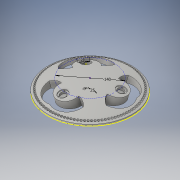
# Autodesk Inventor part: BB-8_headslider_dome
Saved by Autodesk Inventor 2016 (Build 200138000, 138)
## iProperties
Created: 2018-07-20
Part Number: BB-8_headslider_dome
Material: Generic
Document SubType Name: Modeling
Designer: Karcsi
Density: 1 g/cm^3
Appearance: Default
Author: Karcsi
Autodesk Inventor part; units mm, degrees
sketch "Sketch1" plane through (0, 0, 0) normal (0, 0, 1) x (1, 0, 0)
  arc A0 (0, 254) -> (-118.0215, 224.9154) centre (0, 0) ccw construction
  arc A1 (0, -254) -> (118.0215, 224.9154) centre (0, 0) ccw construction
  line L0 (0, 0) -> (0, 254)
  line L1 (0, 0) -> (0, -254)
  line L2 (-118.0215, 224.9154) -> (0, 224.9154) construction
  arc A2 (-118.0215, 224.9154) -> (0, -254) centre (0, 0) ccw construction
  arc A3 (118.0215, 224.9154) -> (0, 254) centre (0, 0) ccw
  line L3 (0, 224.9154) -> (88.5815, 224.9154) construction
  line L4 (0, 254) -> (0, 224.9154)
  line L5 (101.3234, 224.9154) -> (118.0215, 224.9154) construction
  line L6 (88.5815, 224.9154) -> (101.3234, 224.9154) construction
  line L7 (118.0215, 220.9154) -> (0, 220.9154)
  line L8 (0, 224.9154) -> (0, 220.9154)
  line L9 (118.0215, 224.9154) -> (118.0215, 220.9154)
  dimension "d0" = 508
  dimension "d1" = 236.043
  dimension "d23" = 4
  constraints: 20 end point, 8 point on circle, 4 centre point, 4 horizontal, 3 collinear, 2 point on line, 1 coincident, 1 parallel, 1 perpendicular, 1 vertical
  measures "d0" diameter of A0
  measures "d1" distance of L2.start L5.end
  measures "d23" distance between parallel lines of L3 L7
revolve "Revolution1" add sketch "Sketch1" angle 360 about axis through (0, 0, 0) along (0, 1, 0)
sketch "Sketch8" plane through (0, 220.9154, 0) normal (0, -1, 0) x (1, 0, 0)
  circle A0 centre (0, 0) radius 118.0215 projected
  line L0 (-84.745, -82.1423) -> (-100.1458, -62.4492)
  dimension "d24" = 25
  constraints: 2 end point, 2 point on circle
  measures "d24" distance of L0.start L0.end
ref_plane "Work Plane4" through (-86.2431, 224.9938, -83.3138) normal (0.3329064, -0.9063078, 0.2603451) x (-0.6160289, 0, 0.7877236)
ref_plane "Work Plane3" through (-84.745, 220.9154, -82.1423) normal (0.3329064, -0.9063078, 0.2603451) x (-0.6160289, 0, 0.7877236)
ref_plane "Work Plane5" through (0, 254.2529, 0) normal (0, -1, 0) x (1, 0, 0)
sketch "Sketch10" plane through (-86.2431, 224.9938, -83.3138) normal (0.3329064, -0.9063078, 0.2603451) x (-0.6160289, 0, 0.7877236)
  line L0 (9.3666, -17.4194) -> (9.0029, -1.1358) construction
  ellipse E0 centre (12.5, -108.0527) end of major axis (130.5215, -108.0527) minor radius 106.9638 projected
  circle A0 centre (9.1847, -9.2776) radius 2.75
  point P0 (12.5, -12.9993)
  dimension "d31" = 16.2836
  dimension "d32" = 5.5
  constraints: 2 end point, 1 centre point, 1 midpoint, 2 other
  measures "d31" vertical distance of L0.start L0.end
  measures "d32" diameter of A0
extrude "Extrusion6" cut sketch "Sketch10" along normal blind 8 contours A0
pattern_circular "Circular Pattern1" count 100 over 360 about axis through (0, -10, 0) along (0, 1, 0) of "Extrusion6"
ref_plane "Work Plane7" through (-86.8858, 231.0576, -83.8164) normal (0.2038779, -0.9659258, 0.15944) x (-0.6160289, 0, 0.7877236)
ref_plane "Work Plane6" through (-84.745, 220.9154, -82.1423) normal (0.2038779, -0.9659258, 0.15944) x (-0.6160289, 0, 0.7877236)
sketch "Sketch15" plane through (0, 254.2529, 0) normal (0, -1, 0) x (1, 0, 0)
  circle A0 centre (0, 0) radius 70 construction
  dimension "d43" = 140
  constraints: 1 centre point, 1 coincident
  measures "d43" diameter of A0
sketch "Sketch16" plane through (-86.8858, 231.0576, -83.8164) normal (0.2038779, -0.9659258, 0.15944) x (-0.6160289, 0, 0.7877236)
  ellipse E0 centre (12.5, -121.9872) end of major axis (82.5, -121.9872) minor radius 67.6148 projected
  line L0 (12.5, -298.4228) -> (12.5, 63.3053)
  line L1 (12.5, -258.4808) -> (-169.7544, -258.4808)
  line L2 (12.5, -258.4808) -> (193.6614, -258.4808)
  circle A0 centre (12.5, -54.3724) radius 12.5
  point P0 (12.5, -56.1817)
  dimension "d44" = 182.2544
  dimension "d45" = 181.1614
  dimension "d46" = 25
  constraints: 6 end point, 2 horizontal, 2 point on line, 1 centre point, 1 vertical, 1 vertical alignment, 1 other
  measures "d44" distance of L1.start L1.end
  measures "d45" distance of L1.start L2.end
  measures "d46" diameter of A0
sketch "Sketch17" plane through (-86.8858, 231.0576, -83.8164) normal (0.2038779, -0.9659258, 0.15944) x (-0.6160289, 0, 0.7877236)
  circle A0 centre (12.5, -54.3724) radius 8.5
  point P0 (12.5, -56.1817)
  dimension "d47" = 17
  constraints: 1 centre point, 1 coincident
  measures "d47" diameter of A0
extrude "Extrusion7" cut sketch "Sketch16" along normal blind 3 contours A0 L0 E0 | E0 L0 A0 | L0 A0 E0 | E0 A0 L0 picked at (13.5203, -62.5789) picked at (14.4702, -50.3327) picked at (11.4797, -62.5789) picked at (10.4798, -50.3445)
extrude "Extrusion8" cut sketch "Sketch17" along normal blind 9
pattern_circular "Circular Pattern2" count 3 over 360 about axis through (0, -10, 0) along (0, 1, 0) of "Extrusion8", "Extrusion7"
sketch "Sketch18" plane through (-52.6035, 242.2324, -41.1379) normal (-0.2038779, 0.9659258, -0.15944) x (0.9784424, 0.2065197, 0)
  point P0 (1.4437, -1.0906)
sketch "Sketch20" plane through (0, 220.9154, 0) normal (0, -1, 0) x (1, 0, 0)
  line L0 (12.5, 4.5) -> (-12.5, 4.5)
  line L1 (-12.5, 4.5) -> (-12.5, -4.5)
  line L2 (-12.5, -4.5) -> (12.5, -4.5)
  line L3 (12.5, -4.5) -> (12.5, 4.5)
  point P0 (0, 0)
  dimension "d60" = 25
  dimension "d61" = 9
  constraints: 8 end point, 2 parallel, 1 horizontal, 1 perpendicular
  measures "d60" distance of L2.end L1.end
  measures "d61" distance of L1.end L0.end
sketch "Sketch21" plane through (0, 220.9154, 0) normal (0, -1, 0) x (1, 0, 0)
  line L0 (12.5, -4.5) -> (12.5, 4.5) projected
  line L1 (-12.5, -4.5) -> (12.5, -4.5) projected
  line L2 (-12.5, 4.5) -> (-12.5, -4.5) projected
  line L3 (12.5, 4.5) -> (-12.5, 4.5) projected
  line L4 (12.5, -4.5) -> (-12.5, -4.5)
  line L5 (-12.5, -4.5) -> (-12.5, -12.5)
  line L6 (-12.5, -12.5) -> (12.5, -12.5)
  line L7 (12.5, -12.5) -> (12.5, -4.5)
  line L8 (12.5, 4.5) -> (-12.5, 4.5)
  line L9 (-12.5, 4.5) -> (-12.5, 12.5)
  line L10 (-12.5, 12.5) -> (12.5, 12.5)
  line L11 (12.5, 12.5) -> (12.5, 4.5)
  point P0 (0, 0)
  dimension "d62" = 8
  dimension "d63" = 8
  constraints: 16 end point, 4 parallel, 2 horizontal, 2 perpendicular, 1 point on line
  measures "d62" distance of L5.end L4.end
  measures "d63" distance of L8.end L9.end
extrude "Extrusion9" cut sketch "Sketch21" against normal blind 0.2 contours L7 L6 L5 L1 | L3 L9 L10 L11
sketch "Sketch22" plane through (12.5, 220.9154, -12.5) normal (0, 0, 1) x (-1, 0, 0)
  circle A0 centre (12.5, -12.5) radius 12.5
  circle A1 centre (12.5, -12.5) radius 1.5
  point P0 (12.5, 220.9154)
  dimension "d66" = 25
  dimension "d67" = 3
  constraints: 2 centre point, 1 coincident
  measures "d66" diameter of A0
  measures "d67" diameter of A1
extrude "Extrusion11" cut sketch "Sketch22" against normal blind 30 contours A1
sketch "Sketch26" plane through (61.9282, 242.2324, -24.987) normal (0.240018, 0.9659258, -0.0968434) x (0.9704875, -0.2411515, 0)
  circle A0 centre (0, 0) radius 12.5 projected
  circle A1 centre (0, 0) radius 8.5 projected
  circle A2 centre (10, 0) radius 1
  circle A3 centre (-5, 8.6603) radius 1
  circle A4 centre (-5, -8.6603) radius 1
  point P0 (-1.6858, -0.657)
  dimension "d76" = 2
  dimension "d79" = 360
  constraints: 3 centre point, 7 other
  measures "d76" diameter of A2
hole "Hole1" at (71.6331, 239.8209, -24.987) at (56.8735, 242.6242, -33.6066) at (57.278, 244.2521, -16.3675) direction (-0.240018, -0.9659258, 0.0968434) diameter 2 depth 10 tip angle 118
pattern_circular "Circular Pattern3" count 3 over 360 about axis through (0, -10, 0) along (0, 1, 0) of "Hole1"
sketch "Sketch38" plane through (-86.8858, 231.0576, -83.8164) normal (0.2038779, -0.9659258, 0.15944) x (-0.6160289, 0, 0.7877236)
  arc A0 (12.5, -19.454) -> (-43.8881, -61.2033) centre (-0.0547, -61.4517) ccw
  line L0 (12.5, -56.1817) -> (12.5, -19.454) construction
  arc A1 (68.8881, -61.2033) -> (12.5, -19.454) centre (25.0547, -61.4517) ccw
  arc A2 (-43.8881, -61.2033) -> (-15.6918, -72.5813) centre (-18.4468, -38.7824) ccw
  arc A3 (40.6918, -72.5813) -> (68.8881, -61.2033) centre (43.4468, -38.7824) ccw
  arc A4 (40.6918, -72.5813) -> (-15.6918, -72.5813) centre (12.5, -65.4459) ccw
  constraints: 10 point on circle, 5 centre point, 4 symmetric about line, 2 end point, 1 vertical, 2 other
extrude "Extrusion19" cut sketch "Sketch38" along normal blind 82.3875
pattern_circular "Circular Pattern4" count 3 over 360 about axis through (0, -10, 0) along (0, 1, 0) of "Extrusion19"
sketch "Sketch43" plane through (0, 220.9154, 0) normal (0, -1, 0) x (1, 0, 0)
  line L0 (12.5, 4.5) -> (-12.5, 4.5) projected
  line L1 (-12.5, 12.5) -> (12.5, 12.5) projected
  line L2 (-12.5, 4.5) -> (12.5, 4.5)
  line L3 (12.5, 4.5) -> (12.5, 12.5)
  line L4 (12.5, 12.5) -> (-12.5, 12.5)
  line L5 (-12.5, 12.5) -> (-12.5, 4.5)
  line L6 (12.5, -12.5) -> (-12.5, -12.5) projected
  line L7 (-12.5, -4.5) -> (12.5, -4.5)
  line L8 (12.5, -4.5) -> (12.5, -12.5)
  line L9 (12.5, -12.5) -> (-12.5, -12.5)
  line L10 (-12.5, -12.5) -> (-12.5, -4.5)
  point P0 (0, 0)
  constraints: 16 end point, 4 parallel, 2 horizontal, 2 perpendicular
extrude "Extrusion22" add sketch "Sketch43" along normal blind 25
sketch "Sketch44" plane through (12.5, 220.9154, -12.5) normal (0, 0, -1) x (-1, 0, 0)
  circle A0 centre (12.5, -12.5) radius 12.5
  circle A1 centre (12.5, -12.5) radius 1.5
  point P0 (12.5, -220.9154)
  dimension "d118" = 25
  dimension "d119" = 3
  constraints: 2 centre point, 1 coincident
  measures "d118" diameter of A0
  measures "d119" diameter of A1
extrude "Extrusion23" cut sketch "Sketch44" against normal blind 25 contours A1
fillet "Fillet2" radius 2 8 edges at (12.5, 195.9154, 8.5) (0, 195.9154, 12.5) (-12.5, 195.9154, 8.5) (0, 195.9154, 4.5) (0, 195.9154, -4.5) (0, 195.9154, -12.5) (-12.5, 195.9154, -8.5) (12.5, 195.9154, -8.5)
body "Solid1"
